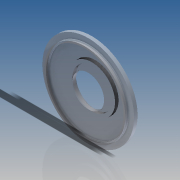
# Autodesk Inventor part: 99542-MilkyWhite
Saved by Autodesk Inventor 2016 SP2 (Build 200236200, 236)
## iProperties
Created: 2015-09-01
Part Number: 99542-MilkyWhite
Material: ABS Plastic
Document SubType Name: Modeling
Designer: D. Kohfeld
Mass: 0.295494 g
Surface Area: 8.07666 cm^2
Volume: 0.278768 cm^3
Density: 1.06 g/cm^3
Appearance: MilkyWhite
Author: D. Kohfeld
Autodesk Inventor part; units mm, degrees
ref_plane "YZ Plane" through (0, 0, 0) normal (1, 0, 0) x (0, 1, 0)
ref_plane "XZ Plane" through (0, 0, 0) normal (0, 1, 0) x (-1, 0, 0)
ref_plane "XY Plane" through (0, 0, 0) normal (0, 0, 1) x (1, 0, 0)
sketch "Sketch2" plane through (0, 0, 0) normal (0, 1, 0) x (-1, 0, 0)
  line L0 (0, 0.8) -> (0, -0.8)
  line L1 (3.6, 0.8) -> (3.6, 0)
  line L2 (3.6, 0) -> (4.4, 0)
  line L3 (4.4, 0) -> (4.4, -0.8)
  line L4 (4.4, -0.8) -> (5.28, -0.8)
  line L5 (5.28, -0.8) -> (5.28, 0)
  line L6 (5.28, 0) -> (10.4, 0)
  line L7 (10.4, 0) -> (10.4, 0.8)
  line L8 (10.4, 0.8) -> (9.2, 0.8)
  line L9 (9.2, 0.8) -> (9.2, 1.6)
  line L10 (9.2, 1.6) -> (8.8, 1.6)
  line L11 (8.8, 1.6) -> (8.8, 0.8)
  line L12 (8.8, 0.8) -> (3.6, 0.8)
  point P0 (0, 0)
  point P1 (0, 0)
  dimension "d0" = 8.8
  dimension "d1" = 10.56
  dimension "d2" = 0.8
  dimension "d3" = 20.8
  dimension "d5" = 0.8
  dimension "d6" = 7.2
  dimension "d7" = 18.4
  dimension "d8" = 17.6
  dimension "d9" = 0.8
  constraints: 26 end point, 7 vertical, 6 horizontal, 4 horizontal alignment, 1 coincident, 1 midpoint
  measures "d0" diameter of L3 L0
  measures "d1" diameter of L5 L0
  measures "d2" distance between parallel lines of L4 L6
  measures "d3" diameter of L7 L0
  measures "d5" distance from line of L1.start L2
  measures "d6" diameter of L1 L0
  measures "d7" diameter of L9 L0
  measures "d8" diameter of L11 L0
  measures "d9" distance between parallel lines of L10 L8
revolve "Revolution1" add sketch "Sketch2" angle 360 about axis through (0, 0, 0.8) along (0, 0, -1)
equation "\"d6\" = tlad"
equation "\"tlad\" = 7.2"
body "Solid1"
